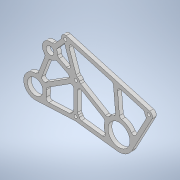
# Autodesk Inventor part: ギア抑え
Saved by Autodesk Inventor 2022.2 (Build 262287010, 287A)
## iProperties
Created: 2022-01-29
Part Number: ギア抑え
Material: Generic
Document SubType Name: Modeling
Designer: acps
Density: 1 g/cm^3
Appearance: Default
Author: acps
Autodesk Inventor part; units mm, degrees
ref_plane "YZ Plane" through (0, 0, 0) normal (1, 0, 0) x (0, 1, 0)
ref_plane "XZ Plane" through (0, 0, 0) normal (0, 1, 0) x (-1, 0, 0)
ref_plane "XY Plane" through (0, 0, 0) normal (0, 0, 1) x (1, 0, 0)
sketch "Sketch2" plane through (0, 0, 0) normal (0, 0, 1) x (1, 0, 0)
  circle A0 centre (58.3063, 43.4) radius 1.25
  circle A1 centre (46.4683, 30) radius 3
  circle A2 centre (35, 0) radius 6.025
  circle A3 centre (66.4734, 20) radius 1.25
  circle A4 centre (66.4734, 20) radius 3
  circle A5 centre (66.299, -4.4994) radius 1.25
  circle A6 centre (58.3063, 43.4) radius 3
  circle A7 centre (66.299, -4.4994) radius 3
  circle A8 centre (46.4683, 30) radius 6
  circle A9 centre (100, 0) radius 8.525
  circle A10 centre (123.045, 25) radius 1.25
  circle A11 centre (123.045, 25) radius 3
  circle A12 centre (100, 0) radius 11.525
  circle A13 centre (35, 0) radius 9.025
  line L0 (59.1265, 46.2857) -> (123.8652, 27.8857)
  line L1 (61.192, 42.5798) -> (120.1593, 25.8202)
  line L2 (125.6902, 23.5847) -> (110.1618, -5.4372)
  line L3 (121.6297, 22.3548) -> (111.1756, 2.8165)
  line L4 (100.4881, 11.5147) -> (98.6843, 31.9238)
  line L5 (97.4998, 11.2505) -> (95.595, 32.8018)
  line L6 (67.9362, 17.3808) -> (67.9547, 17.3697) construction
  line L7 (69.4731, 19.9572) -> (90.955, 7.1424)
  line L8 (66.4734, 20) -> (100, 0) construction
  line L9 (66.4734, 20) -> (123.045, 25) construction
  line L10 (105.736, 12.0769) -> (89.9353, 10.6804) construction
  line L11 (100, 0) -> (96.8569, 35.562) construction
  line L12 (65.9378, -7.4775) -> (66.3598, -7.5287) construction
  line L13 (35.4415, -9.0142) -> (66.0211, -7.5166)
  arc A14 (66.3598, -7.5287) -> (66.0211, -7.5166) centre (66.119, -9.5142) ccw
  line L14 (66.3598, -7.5287) -> (98.6121, -11.4411)
  line L15 (66.0211, -7.5166) -> (66.4458, -7.4958) construction
  line L16 (91.2742, -7.529) -> (69.2772, -4.8606)
  line L17 (42.006, -5.6891) -> (63.3026, -4.6461)
  line L18 (64.955, 17.4127) -> (64.9539, 17.2571) construction
  line L19 (67.8175, -1.912) -> (67.9299, 13.8769)
  line L20 (66.4734, 20) -> (66.299, -4.4994) construction
  arc A15 (70.9544, 15.5803) -> (67.9299, 13.8769) centre (69.9298, 13.8627) ccw
  line L21 (67.9547, 17.3697) -> (67.9549, 17.3913) construction
  line L22 (67.9547, 17.3697) -> (70.9544, 15.5803) construction
  line L23 (35, 0) -> (46.4683, 30) construction
  line L24 (42.9928, 25.1091) -> (36.7767, 8.8484)
  line L25 (39.5789, 7.7772) -> (45.795, 24.0379)
  line L26 (46.4683, 30) -> (66.4734, 20) construction
  line L27 (50.994, 26.0607) -> (60.2686, 21.4247)
  line L28 (52.3354, 28.7442) -> (59.4344, 25.1956)
  line L29 (60.5787, 41.4413) -> (67.0335, 22.9473)
  line L30 (66.4734, 20) -> (58.3063, 43.4) construction
  line L31 (57.7462, 40.4527) -> (62.2169, 27.6436)
  arc A16 (59.4344, 25.1956) -> (62.2169, 27.6436) centre (60.3286, 26.9845) ccw
  line L32 (62.2169, 27.6436) -> (64.2011, 21.9587) construction
  line L33 (59.4344, 25.1956) -> (64.8202, 22.5034) construction
  line L34 (70.9544, 15.5803) -> (89.418, 4.566)
  line L35 (67.9299, 13.8769) -> (67.9547, 17.3697) construction
  line L36 (46.4683, 30) -> (58.3063, 43.4) construction
  line L37 (51.4388, 33.3607) -> (57.7104, 40.4598)
  line L38 (49.1905, 35.3469) -> (55.462, 42.446)
  arc A17 (58.8599, 37.2619) -> (55.4728, 37.927) centre (56.9716, 36.6028) ccw
  line L39 (35, 0) -> (66.4734, 20) construction
  line L40 (41.7067, 6.0391) -> (60.447, 17.9477)
  line L41 (65.0851, 17.3406) -> (61.8551, 15.288) construction
  arc A18 (60.447, 17.9477) -> (60.2686, 21.4247) centre (59.3743, 19.6357) ccw
  line L42 (60.2686, 21.4247) -> (63.4788, 19.8199) construction
  line L43 (60.447, 17.9477) -> (63.4761, 19.8726) construction
  arc A19 (64.9277, 13.5858) -> (61.8551, 15.288) centre (62.9278, 13.6) ccw
  line L44 (61.8551, 15.288) -> (43.3157, 3.507)
  line L45 (64.9277, 13.5858) -> (64.8176, -1.8907)
  line L46 (64.9539, 17.2571) -> (64.9277, 13.5858) construction
  point P0 (0, 0)
  point P1 (63.4788, 19.8199)
  point P2 (64.8119, -2.686)
  point P3 (47.0701, 27.061)
  point P4 (48.1215, 27.4966)
  point P5 (63.8273, 22.9997)
  point P6 (49.4629, 30.1801)
  point P7 (49.3126, 30.954)
  point P8 (57.7343, 40.4869)
  point P9 (63.8353, 23.0067)
  point P10 (69.4731, 19.9572)
  point P11 (67.0335, 22.9473)
  point P12 (60.6742, 41.1676)
  point P13 (120.1358, 24.2674)
  point P14 (120.1812, 24.1064)
  point P15 (100.658, 2.927)
  point P16 (98.5372, 2.6192)
  point P17 (95.5346, 0.9171)
  point P18 (67.8113, -2.7842)
  point P19 (67.9547, 17.3697)
  point P20 (47.0643, 32.9402)
  point P21 (44.2209, 28.0127)
  point P22 (66.0689, -5.9816)
  point P23 (66.4975, -5.9862)
  point P24 (97.6233, -1.8306)
  point P25 (102.8638, 0.8936)
  point P26 (122.387, 22.073)
  point P27 (120.956, 27.1531)
  point P28 (61.2155, 44.1326)
  point P29 (55.462, 42.446)
  point P30 (99.2315, -1.2882)
  point P31 (99.2644, 1.4151)
  point P32 (100.7685, 1.2882)
  point P33 (65.8027, 18.6583)
  point P34 (65.705, 18.7118)
  point P35 (67.1441, 21.3417)
  point P36 (45.3441, 30.9931)
  point P37 (47.139, 31.3417)
  point P38 (47.7709, 29.2089)
  point P39 (62.6167, 23.75)
  point P40 (63.8469, 21.7439)
  point P41 (63.7276, 4.995)
  point P42 (48.9428, 29.7841)
  point P43 (49.819, 30.1472)
  point P44 (62.9071, 26.3997)
  point P45 (50.9368, 32.3834)
  point P46 (50.8115, 33.0283)
  point P47 (57.8297, 40.9724)
  point P48 (62.9138, 26.4056)
  point P49 (67.612, 23.8643)
  point P50 (65.579, 26.356)
  point P51 (60.2796, 41.5397)
  point P52 (109.8309, 27.4562)
  point P53 (109.8687, 27.322)
  point P54 (93.5994, 9.6725)
  point P55 (91.8321, 9.416)
  point P56 (89.3299, 7.9976)
  point P57 (66.2271, 4.9132)
  point P58 (66.3467, 21.7081)
  point P59 (48.9379, 34.6835)
  point P60 (46.5685, 30.5773)
  point P61 (64.7751, 2.2487)
  point P62 (65.1323, 2.2448)
  point P63 (91.0705, 5.7078)
  point P64 (95.4376, 7.978)
  point P65 (111.7069, 25.6275)
  point P66 (110.5144, 29.861)
  point P67 (60.7307, 44.0105)
  point P68 (55.9361, 42.605)
  point P69 (92.4107, 6.1598)
  point P70 (92.438, 8.4126)
  point P71 (93.6914, 8.3068)
  point P72 (64.5533, 22.7819)
  point P73 (64.4718, 22.8265)
  point P74 (65.6711, 25.0181)
  point P75 (47.5045, 33.0609)
  point P76 (49.0002, 33.3514)
  point P77 (49.5268, 31.5741)
  dimension "d81" = 6
  dimension "d77" = 2.5
  dimension "d78" = 6
  dimension "d79" = 12.05
  dimension "d80" = 2.5
  dimension "d82" = 2.5
  dimension "d83" = 6
  dimension "d84" = 6
  dimension "d85" = 3
  dimension "d86" = 17.05
  dimension "d87" = 2.5
  dimension "d88" = 6
  dimension "d89" = 3
  dimension "d90" = 3
  dimension "d91" = 3
  dimension "d92" = 3
  dimension "d93" = 3
  dimension "d94" = 3
  dimension "d95" = 1.5
  dimension "d96" = 1.5
  dimension "d97" = 2
  dimension "d98" = 3
  dimension "d99" = 3
  dimension "d100" = 3
  dimension "d101" = 1.5
  dimension "d102" = 2
  dimension "d103" = 3
  dimension "d104" = 1.5
  dimension "d105" = 3
  dimension "d106" = 1.5
  dimension "d107" = 3
  dimension "d108" = 1.5
  dimension "d109" = 2
  dimension "d110" = 3
  dimension "d111" = 1.5
  dimension "d112" = 2
  dimension "d113" = 3
  dimension "d114" = 1.5
  dimension "d115" = 2
  dimension "d116" = 2
  constraints: 94 end point, 42 parallel, 40 point on circle, 34 tangent, 18 centre point, 11 coincident, 7 point on line, 2 perpendicular, 33 other
  measures "d77" diameter of A0
  measures "d78" diameter of A1
  measures "d79" diameter of A2
  measures "d80" diameter of A3
  measures "d82" diameter of A5
  measures "d83" diameter of A6
  measures "d84" diameter of A7
  measures "d85" radial gap between concentric circles of A1 A8
  measures "d86" diameter of A9
  measures "d87" diameter of A10
  measures "d88" diameter of A11
  measures "d90" radial gap between concentric circles of A2 A13
  measures "d91" distance between parallel lines of L1 L0
  measures "d92" distance between parallel lines of L2 L3
  measures "d93" distance between parallel lines of L4 L5
  measures "d94" distance between parallel lines of L6 L7
  measures "d95" distance between parallel lines of L7 L8
  measures "d96" distance between parallel lines of L11 L5
  measures "d97" radius of A14
  measures "d98" distance between parallel lines of L14 L16
  measures "d99" distance between parallel lines of L13 L17
  measures "d100" distance between parallel lines of L18 L19
  measures "d101" distance between parallel lines of L18 L20
  measures "d102" radius of A15
  measures "d103" distance between parallel lines of L24 L25
  measures "d104" distance between parallel lines of L23 L25
  measures "d105" distance between parallel lines of L27 L28
  measures "d106" distance between parallel lines of L27 L26
  measures "d107" distance between parallel lines of L31 L29
  measures "d108" distance between parallel lines of L29 L30
  measures "d109" radius of A16
  measures "d110" distance between parallel lines of L38 L37
  measures "d111" distance between parallel lines of L36 L37
  measures "d112" radius of A17
  measures "d113" distance between parallel lines of L40 L41
  measures "d114" distance between parallel lines of L41 L39
  measures "d115" radius of A18
  measures "d116" radius of A19
extrude "Extrusion1" add sketch "Sketch2" against normal blind 3 contours A4 | A4 L7 A12 L34 A15 L19 A7 L45 A19 L44 A13 L40 A18 L27 A8 L28 A16 L31 A6 L29 | A6 | A12 | A6 L0 A11 L1 | L5 L1 L4 A12 | L37 A8 L38 A6 | A12 L14 A14 L13 A13 L17 A7 L16 | L3 A11 L2 A12 | A7 | A8 | A11 | A8 L25 A13 L24 | A13
fillet "Fillet2" radius 2 30 edges at (121.6297, 22.3548, -1.5) (120.1593, 25.8202, -1.5) (90.955, 7.1424, -1.5) (100.4881, 11.5147, -1.5) (111.1756, 2.8165, -1.5) (69.2772, -4.8606, -1.5) (97.4998, 11.2505, -1.5) (95.595, 32.8018, -1.5) (89.418, 4.566, -1.5) (64.8176, -1.8907, -1.5) (63.3026, -4.6461, -1.5) (91.2742, -7.529, -1.5) (67.8175, -1.912, -1.5) (43.3157, 3.507, -1.5) (42.006, -5.6891, -1.5) (39.5789, 7.7772, -1.5) (41.7067, 6.0391, -1.5) (52.3354, 28.7442, -1.5) (67.0335, 22.9473, -1.5) (69.4731, 19.9572, -1.5) (60.5787, 41.4413, -1.5) (61.192, 42.5798, -1.5) (57.7462, 40.4527, -1.5) (50.994, 26.0607, -1.5) (45.795, 24.0379, -1.5) (42.9928, 25.1091, -1.5) (49.1905, 35.3469, -1.5) (55.462, 42.446, -1.5) (36.7767, 8.8484, -1.5) (98.6843, 31.9238, -1.5)
body "Solid1"
